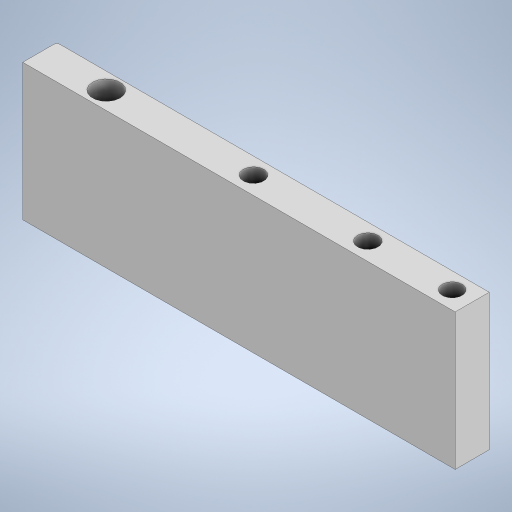
# Autodesk Inventor part: BASE
Saved by Autodesk Inventor 2024 (Build 280153000, 153)
## iProperties
Created: 2023-10-23
Part Number: BASE
Material: Generic
Document SubType Name: Modeling
Designer: tinas
Density: 1 g/cm^3
Appearance: Default
Author: tinas
Autodesk Inventor part; units mm, degrees
ref_plane "YZ Plane" through (0, 0, 0) normal (1, 0, 0) x (0, 1, 0)
ref_plane "XZ Plane" through (0, 0, 0) normal (0, 1, 0) x (-1, 0, 0)
ref_plane "XY Plane" through (0, 0, 0) normal (0, 0, 1) x (1, 0, 0)
sketch "Sketch1" plane through (0, 0, 0) normal (0, 1, 0) x (-1, 0, 0)
  line L0 (0, 0) -> (317, 0)
  line L1 (317, 0) -> (317, 25)
  line L2 (317, 25) -> (0, 25)
  line L3 (0, 25) -> (0, 0)
  dimension "d0" = 317
  dimension "d1" = 25
  constraints: 8 end point, 2 parallel, 1 horizontal, 1 perpendicular
  measures "d0" distance of L1.end L2.end
  measures "d1" distance of L0.end L1.end
extrude "Extrusion1" add sketch "Sketch1" along normal blind 100
fillet "Face Fillet1" radius 2 1 edges at (-317, 50, 0)
sketch "Sketch5" plane through (0, 0, 0) normal (0, 1, 0) x (-1, 0, 0)
  circle A0 centre (15.133, 12.0626) radius 7.2608
  circle A1 centre (76.981, 12.0626) radius 7.5
  circle A2 centre (160.761, 12.0626) radius 7.5
  circle A3 centre (268.666, 12.0626) radius 10.0887
  point P0 (0, 0)
  dimension "d16" = 15
  dimension "d17" = 15
  constraints: 4 centre point
  measures "d16" diameter of A1
  measures "d17" diameter of A2
extrude "Extrusion4" cut sketch "Sketch5" along normal blind 100
body "Solid1"
